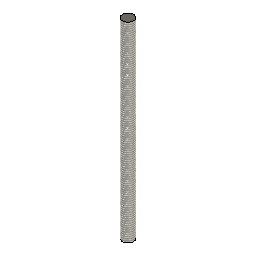
Avionics Bay (Autodesk Fusion 360 archive; units mm, degrees)
design "M6x90mm Threaded Rod"
part number: 2026-03-08-09-04-35-086
Autodesk Fusion 360 part; units mm, degrees
sketch "Sketch1" plane through (0, 0, 0) normal (0, 0, 1) x (1, 0, 0)
  circle A0 centre (0, 0) radius 3
  dimension "d1" = 6
  constraint coincident A0.centre origin
  measures "d1" diameter of A0
extrude "Extrude1" add sketch "Sketch1" along normal blind 100
thread "Thread1" "ISO Metric profile 6.0 M6x1 M6x1 6g" major diameter 5.884 minor diameter 4.7435 pitch 1 angle 60 resizes the face on face at (2.9851, -0.2987, 33.3333)

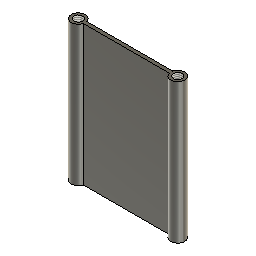
design "Sled"
part number: 2026-03-08-09-11-17-027
Autodesk Fusion 360 part; units mm, degrees
sketch "Sketch1" plane through (0, 0, 0) normal (0, 0, 1) x (1, 0, 0)
  circle A0 centre (-28.5, 0) radius 4
  circle A1 centre (28.5, 0) radius 4
  line L0 (-24.627, 1) -> (24.627, 1)
  line L1 (-24.627, -1) -> (24.627, -1)
  dimension "d1" = 8
  dimension "d2" = 28.5
  dimension "d3" = 8
  dimension "d4" = 28.5
  dimension "d5" = 1
  dimension "d6" = 1
  constraint coincident A0 L0.start
  constraint coincident A1 L0.end
  constraint horizontal L0
  constraint coincident A0 L1.start
  constraint coincident A1 L1.end
  constraint parallel L0 L1
  measures "d1" diameter of A0
  measures "d2" distance of origin A0.centre
  measures "d3" diameter of A1
  measures "d4" distance of origin A1.centre
  measures "d5" distance of origin L0
  measures "d6" distance of origin L1
extrude "Extrude1" add sketch "Sketch1" along normal blind 80
sketch "Sketch2" plane through (0, 0, 80) normal (0, 0, 1) x (-1, 0, 0)
  arc A0 (24.627, -1) -> (24.627, 1) centre (28.5, 0) ccw
  line L0 (24.627, 1) -> (-24.627, 1)
  arc A1 (-24.627, 1) -> (-24.627, -1) centre (-28.5, 0) ccw
  line L1 (-24.627, -1) -> (24.627, -1)
  circle A2 centre (28.5, 0) radius 3.1
  circle A3 centre (-28.5, 0) radius 3.1
  dimension "d9" = 6.2
  dimension "d10" = 6.2
  constraint concentric A0 A2
  constraint concentric A1 A3
  measures "d9" diameter of A2
  measures "d10" diameter of A3
extrude "Extrude2" cut sketch "Sketch2" against normal blind 90 contours A2 | A3
thread "Thread1" "ISO Metric profile 6.0 M6x1 M6x1 6H" major diameter 6.147 minor diameter 5.035 pitch 1 angle 60 resizes the face on face at (-31.5846, 0.3087, 53.3333)
thread "Thread2" "ISO Metric profile 6.0 M6x1 M6x1 6H" major diameter 6.147 minor diameter 5.035 pitch 1 angle 60 resizes the face on face at (25.4154, 0.3087, 53.3333)
